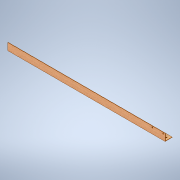
# Autodesk Inventor part: Angulo 2020x450
Saved by Autodesk Inventor 2021 (Build 250183000, 183)
## iProperties
Created: 2023-01-27
Part Number: Angulo 2020x450
Material: Madera (cerezo)
Document SubType Name: Modeling
Designer: Diego.labarca
Density: 0.63 g/cm^3
Appearance: Cerezo - Natural brillo bajo
Author: Diego.labarca
Autodesk Inventor part; units mm, degrees
ref_plane "YZ Plane" through (0, 0, 0) normal (1, 0, 0) x (0, 1, 0)
ref_plane "XZ Plane" through (0, 0, 0) normal (0, 1, 0) x (-1, 0, 0)
ref_plane "XY Plane" through (0, 0, 0) normal (0, 0, 1) x (1, 0, 0)
sketch "Boceto1" plane through (0, 0, 0) normal (1, 0, 0) x (0, 1, 0)
  line L0 (0, 0) -> (20, 0)
  line L1 (20, 0) -> (20, -1)
  line L2 (20, -1) -> (0, -1)
  line L3 (0, -1) -> (0, 0)
  line L4 (0, 0) -> (1, 0)
  line L5 (1, 0) -> (1, -20)
  line L6 (1, -20) -> (0, -20)
  line L7 (0, -20) -> (0, 0)
  point P0 (1, -1)
  dimension "d0" = 20
  dimension "d1" = 20
  dimension "d2" = 1
  dimension "d3" = 1
  constraints: 16 end point, 4 parallel, 2 horizontal, 2 perpendicular
  measures "d0" distance of L6.end L0.start
  measures "d1" distance of L0.start L0.end
  measures "d2" distance of L5.end L6.end
  measures "d3" distance of L0.end L1.end
extrude "Extrusión1" add sketch "Boceto1" along normal blind 450
sketch "Boceto2" plane through (0, 1, -1) normal (0, 0, -1) x (-1, 0, 0)
  circle A0 centre (-444.35, 15.65) radius 1.75
  line L0 (0, 19) -> (-450, 19) projected
  line L1 (-450, 0) -> (-450, 19) projected
  circle A1 centre (-413.35, 15.65) radius 1.75
  point P0 (0, -1)
  dimension "d6" = 3.5
  dimension "d7" = 3.35
  dimension "d8" = 5.65
  dimension "d11" = 3.5
  dimension "d12" = 31
  dimension "d13" = 3.35
  constraints: 2 centre point
  measures "d6" diameter of A0
  measures "d7" distance from line of L0 A0.centre
  measures "d8" distance from line of L1 A0.centre
  measures "d11" diameter of A1
  measures "d12" distance of A0.centre A1.centre
  measures "d13" distance from line of L0 A1.centre
extrude "Extrusión2" cut sketch "Boceto2" against normal through all
sketch "Boceto3" plane through (0, 1, -1) normal (0, 1, 0) x (1, 0, 0)
  circle A0 centre (443, 10) radius 1.5
  circle A1 centre (417, 10) radius 1.5
  line L0 (0, 19) -> (450, 19) projected
  line L1 (450, 19) -> (450, 0) projected
  point P0 (0, -1)
  dimension "d14" = 3
  dimension "d15" = 3
  dimension "d16" = 9
  dimension "d17" = 9
  dimension "d18" = 7
  dimension "d19" = 26
  constraints: 2 centre point
  measures "d14" diameter of A0
  measures "d15" diameter of A1
  measures "d16" distance from line of L0 A0.centre
  measures "d17" distance from line of L0 A1.centre
  measures "d18" distance from line of L1 A0.centre
  measures "d19" distance of A0.centre A1.centre
extrude "Extrusión3" cut sketch "Boceto3" against normal through all
equation "\"d1\" = d0"
equation "\"d3\" = d2"
equation "\"d11\" = d6"
equation "\"d13\" = d7"
equation "\"d15\" = d14"
equation "\"d17\" = d16"
